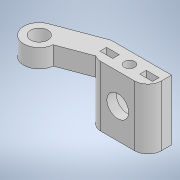
# Autodesk Inventor part: Деталь крепления диска к поворотному механизму
Saved by Autodesk Inventor 2020 (Build 240168000, 168)
## iProperties
Created: 2021-03-15
Part Number: Деталь крепления диска к поворотному механизму
Material: Типовые
Document SubType Name: Modeling
Designer: Антон
Density: 1 g/cm^3
Appearance: По умолчанию
Mass: 2.90777 g
Surface Area: 27.0682 cm^2
Volume: 2.90777 cm^3
Угол_Аккермана: 15,65 град
Высота_сошки: 21,000 мм
Ширина_колесной_базы: 59,900 мм
Длина_колесной_базы: 106,901 мм
Author: Антон
Autodesk Inventor part; units mm, degrees
ref_plane "YZ Plane" through (0, 0, 0) normal (1, 0, 0) x (0, 1, 0)
ref_plane "XZ Plane" through (0, 0, 0) normal (0, 1, 0) x (-1, 0, 0)
ref_plane "XY Plane" through (0, 0, 0) normal (0, 0, 1) x (1, 0, 0)
sketch "Эскиз1" plane through (0, 0, 0) normal (0, 0, 1) x (1, 0, 0)
  line L0 (0, 0) -> (18, 0)
  line L1 (18, 0) -> (18, 18)
  line L2 (18, 18) -> (0, 18)
  line L3 (0, 18) -> (0, 0)
  dimension "d0" = 18
  dimension "d1" = 18
  constraints: 8 end point, 2 parallel, 1 horizontal, 1 perpendicular
  measures "d0" distance of L2.end L1.end
  measures "d1" distance of L1.end L0.end
extrude "Выдавливание1" add sketch "Эскиз1" along normal blind 7
sketch "Эскиз2" plane through (0, 0, 0) normal (0, 0, -1) x (-1, 0, 0)
  line L0 (0, 0) -> (-18, 0) projected
  line L1 (-9, 0) -> (-9, 18)
  line L2 (-18, 18) -> (0, 18) projected
  circle A0 centre (-9, 9) radius 4.025
  dimension "d4" = 8.05
  constraints: 3 midpoint, 2 end point, 1 centre point
  measures "d4" diameter of A0
extrude "Выдавливание2" cut sketch "Эскиз2" against normal blind 4.2
sketch "Эскиз5" plane through (0, 18, 0) normal (0, 1, 0) x (1, 0, 0)
  line L0 (0, 0) -> (18, 0) projected
  line L1 (9, 0) -> (9, -3.5)
  circle A0 centre (9, -3.5) radius 1.55
  dimension "d21" = 3.5
  dimension "d22" = 3.1
  constraints: 2 end point, 1 centre point, 1 coincident, 1 midpoint, 1 vertical
  measures "d21" distance of L1.start L1.end
  measures "d22" diameter of A0
extrude "Выдавливание4" cut sketch "Эскиз5" against normal blind 4
sketch "Эскиз6" plane through (0, 0, 0) normal (0, -1, 0) x (1, 0, 0)
  circle A0 centre (9, 3.5) radius 1.55 projected
  point P0 (0, 0)
  point P1 (7.5329, 7)
  point P2 (10.4671, 7)
  constraints: 1 other
extrude "Выдавливание5" cut sketch "Эскиз6" against normal blind 4
sketch "Эскиз8" plane through (0, 0, 7) normal (0, 0, 1) x (1, 0, 0)
  circle A0 centre (9, 9) radius 4.025 projected
  circle A1 centre (9, 9) radius 4.025 projected
  circle A2 centre (9, 9) radius 3.25
  point P0 (0, 0)
  dimension "d27" = 6.5
  constraints: 1 centre point, 1 coincident
  measures "d27" diameter of A2
extrude "Выдавливание6" cut sketch "Эскиз8" against normal through all contours A2
sketch "Эскиз22" plane through (0, 0, 0) normal (0, 0, -1) x (-1, 0, 0)
  circle A0 centre (-9, 9) radius 4.025 projected
  line L0 (0, 0) -> (-18, 0) projected
  line L1 (0, 18) -> (0, 0) projected
  line L2 (-18, 18) -> (0, 18) projected
  line L3 (-18, 0) -> (-18, 18) projected
  line L4 (-18, 18) -> (-11.8461, 11.8461) construction
  line L5 (0, 18) -> (-6.1539, 11.8461) construction
  line L6 (-18, 0) -> (-11.8461, 6.1539) construction
  line L7 (0, 0) -> (-18, 0) construction
  line L8 (0, 0) -> (-6.1539, 6.1539) construction
  point P0 (-14.9231, 14.9231)
  point P1 (-3.0769, 14.9231)
  point P2 (-3.0769, 3.0769)
  point P3 (-14.9231, 3.0769)
  constraints: 8 end point, 4 midpoint, 4 point on circle, 2 collinear
hole "Отверстие4" at (14.9231, 14.9231, 0) at (3.0769, 14.9231, 0) at (14.9231, 3.0769, 0) at (3.0769, 3.0769, 0) direction (0, 0, 1) diameter 2.2 depth 2.525
sketch "Эскиз23" plane through (0, 0, 0) normal (0, 0, -1) x (-1, 0, 0)
  circle A0 centre (-14.9231, 14.9231) radius 1.1 projected
  line L0 (-16.8231, 16.02) -> (-14.9231, 17.117)
  line L1 (-14.9231, 17.117) -> (-13.0231, 16.02)
  line L2 (-13.0231, 16.02) -> (-13.0231, 13.8261)
  line L3 (-13.0231, 13.8261) -> (-14.9231, 12.7291)
  line L4 (-14.9231, 12.7291) -> (-16.8231, 13.8261)
  line L5 (-16.8231, 13.8261) -> (-16.8231, 16.02)
  circle A1 centre (-3.0769, 14.9231) radius 1.1 projected
  line L6 (-1.1769, 13.8261) -> (-3.0769, 12.7291)
  line L7 (-3.0769, 12.7291) -> (-4.9769, 13.8261)
  line L8 (-4.9769, 13.8261) -> (-4.9769, 16.02)
  line L9 (-4.9769, 16.02) -> (-3.0769, 17.117)
  line L10 (-3.0769, 17.117) -> (-1.1769, 16.02)
  line L11 (-1.1769, 16.02) -> (-1.1769, 13.8261)
  circle A2 centre (-14.9231, 3.0769) radius 1.1 projected
  line L12 (-14.9231, 0.883) -> (-16.8231, 1.98)
  line L13 (-16.8231, 1.98) -> (-16.8231, 4.1739)
  line L14 (-16.8231, 4.1739) -> (-14.9231, 5.2709)
  line L15 (-14.9231, 5.2709) -> (-13.0231, 4.1739)
  line L16 (-13.0231, 4.1739) -> (-13.0231, 1.98)
  line L17 (-13.0231, 1.98) -> (-14.9231, 0.883)
  circle A3 centre (-3.0769, 3.0769) radius 1.1 projected
  line L18 (-4.9769, 1.98) -> (-4.9769, 4.1739)
  line L19 (-4.9769, 4.1739) -> (-3.0769, 5.2709)
  line L20 (-3.0769, 5.2709) -> (-1.1769, 4.1739)
  line L21 (-1.1769, 4.1739) -> (-1.1769, 1.98)
  line L22 (-1.1769, 1.98) -> (-3.0769, 0.883)
  line L23 (-3.0769, 0.883) -> (-4.9769, 1.98)
  line L24 (0, 0) -> (-18, 0) projected
  line L25 (-18, 18) -> (0, 18) projected
  line L26 (-18, 0) -> (-18, 18) projected
  line L27 (0, 18) -> (0, 0) projected
  line L28 (-16.8231, 1.98) -> (-13.0231, 1.98)
  line L29 (-13.0231, 1.98) -> (-13.0231, 0)
  line L30 (-13.0231, 0) -> (-16.8231, 0)
  line L31 (-16.8231, 0) -> (-16.8231, 1.98)
  line L32 (-4.9769, 1.98) -> (-1.1769, 1.98)
  line L33 (-1.1769, 1.98) -> (-1.1769, 0)
  line L34 (-1.1769, 0) -> (-4.9769, 0)
  line L35 (-4.9769, 0) -> (-4.9769, 1.98)
  line L36 (-4.9769, 16.02) -> (-1.1769, 16.02)
  line L37 (-1.1769, 16.02) -> (-1.1769, 18)
  line L38 (-1.1769, 18) -> (-4.9769, 18)
  line L39 (-4.9769, 18) -> (-4.9769, 16.02)
  line L40 (-16.8231, 16.02) -> (-13.0231, 16.02)
  line L41 (-13.0231, 16.02) -> (-13.0231, 18)
  line L42 (-13.0231, 18) -> (-16.8231, 18)
  line L43 (-16.8231, 18) -> (-16.8231, 16.02)
  point P0 (-14.8414, 16.02)
  point P1 (-15.0047, 16.02)
  point P2 (-13.0231, 18)
  point P3 (-16.8231, 0)
  point P4 (-13.0231, 0)
  point P5 (-1.1769, 18)
  point P6 (-4.9769, 18)
  point P7 (-4.9769, 0)
  point P8 (-1.1769, 0)
  dimension "d92" = 3.8
  constraints: 80 end point, 12 parallel, 4 coincident, 4 horizontal, 4 perpendicular, 3 collinear, 3 equal length, 3 point on line, 52 other
  measures "d92" distance between parallel lines of L8 L11
extrude "Выдавливание13" cut sketch "Эскиз23" against normal blind 1.95 from surface at -2.525 contours A0 L40 | A0 L40 L2 L3 L4 L5 | L40 A0 | A0 L40 L0 L1 | L1 L0 L43 L25 L41 | L25 L37 L10 L9 L39 | L36 A1 L11 L6 L7 L8 | L9 L10 L36 A1 | L36 A1 | A1 L36 | L31 L12 L17 L29 L24 | L28 A2 L17 L12 | L13 L14 L15 L16 L28 A2 | L24 L35 L23 L22 L33 | L28 A2 | A2 L28 | L32 A3 L18 L19 L20 L21 | L22 L23 L32 A3 | L32 A3 | A3 L32
sketch "Эскиз24" plane through (0, 18, 0) normal (0, 1, 0) x (1, 0, 0)
  circle A0 centre (9, -3.5) radius 1.55 projected
  circle A1 centre (9, -3.5) radius 1.55 projected
  line L0 (9, -3.5) -> (-12, -9.3835) construction
  line L1 (18, 0) -> (0, 0) projected
  circle A2 centre (-12, -9.3835) radius 2.575
  line L2 (0, 0) -> (0, -7) projected
  line L3 (18, -7) -> (0, -7) projected
  line L4 (-13.6057, -5.0995) -> (0, 0)
  line L5 (0, -7) -> (-7.4431, -9.7897)
  circle A3 centre (-12, -9.3835) radius 4.575
  dimension "Угол_Аккермана" = 15.651
  dimension "d96" = 5.15
  dimension "Высота_сошки" = 21
  dimension "d116" = 9.15
  constraints: 6 end point, 2 centre point, 2 coincident, 2 point on circle, 1 parallel, 1 tangent
  measures "Угол_Аккермана" angle of L1 L0
  measures "d96" diameter of A2
  measures "Высота_сошки" horizontal distance of A0.centre L0.end
  measures "d116" diameter of A3
extrude "Выдавливание14" add sketch "Эскиз24" against normal blind 4 contours L2 L5 A3 L4 | A3
sketch "Эскиз26" plane through (0, 14, 0) normal (0, -1, 0) x (1, 0, 0)
  line L0 (0, 7) -> (-7.4431, 9.7897) projected
  arc A0 (-7.4431, 9.7897) -> (-13.6057, 5.0995) centre (-12, 9.3835) ccw projected
  line L1 (-13.6057, 5.0995) -> (0, 0) projected
  line L2 (0, 7) -> (0, 0) projected
  circle A1 centre (-12, 9.3835) radius 2.575 projected
  point P0 (0, 0)
extrude "Выдавливание16" add sketch "Эскиз26" along normal blind 1.5 contours L2 L1 A0 L0 | A1
fillet "Сопряжение13" radius 4 4 edges at (18, 9, 7) (0, 6.25, 7) (0, 13.25, 7) (0, 16, 7)
equation "\"Ширина_колесной_базы\" = 59.9"
equation "\"Длина_колесной_базы\" = 106.901"
